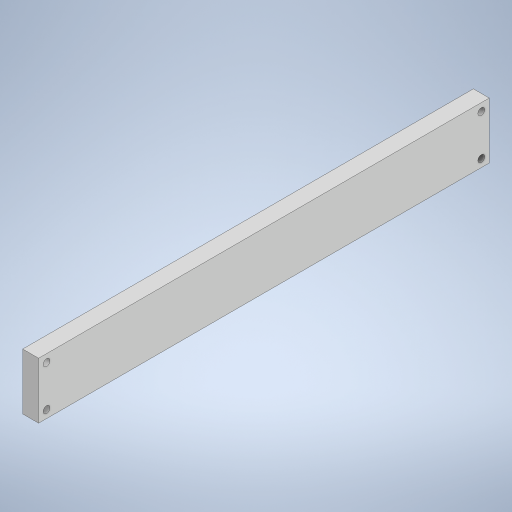
# Autodesk Inventor part: Mold_sideWall
Saved by Autodesk Inventor 2024 (Build 280153000, 153)
## iProperties
Created: 2024-09-09
Part Number: Mold_sideWall
Material: Generic
Document SubType Name: Modeling
Designer: Bruger
Density: 1 g/cm^3
Appearance: Default
Author: Bruger
Autodesk Inventor part; units mm, degrees
ref_plane "YZ Plane" through (0, 0, 0) normal (1, 0, 0) x (0, 1, 0)
ref_plane "XZ Plane" through (0, 0, 0) normal (0, 1, 0) x (-1, 0, 0)
ref_plane "XY Plane" through (0, 0, 0) normal (0, 0, 1) x (1, 0, 0)
sketch "Sketch1" plane through (0, 0, 0) normal (1, 0, 0) x (0, 1, 0)
  line L0 (-12.375, 99.15) -> (12.375, 99.15)
  line L1 (12.375, 99.15) -> (12.375, -99.15)
  line L2 (12.375, -99.15) -> (-12.375, -99.15)
  line L3 (-12.375, -99.15) -> (-12.375, 99.15)
  line L4 (-12.375, 99.15) -> (12.375, -99.15) construction
  line L5 (12.375, 99.15) -> (-12.375, -99.15) construction
  point P0 (0, 0)
  dimension "d0" = 198.3
  dimension "d1" = 24.75
  constraints: 12 end point, 2 midpoint, 2 parallel, 1 horizontal, 1 perpendicular
  measures "d0" distance of L0.end L1.end
  measures "d1" distance between parallel lines of L1 L3
extrude "Extrusion1" add sketch "Sketch1" along normal blind 7
sketch "Sketch2" plane through (7, 0, 0) normal (1, 0, 0) x (0, 0, -1)
  circle A0 centre (-95.65, 8.95) radius 1.5
  line L0 (-99.15, 12.375) -> (-99.15, -12.375) projected
  line L1 (99.15, 12.375) -> (-99.15, 12.375) projected
  line L2 (-113.68, 5.525) -> (-113.68, 12.375)
  point P0 (0, 0)
  dimension "d4" = 3.5
  dimension "d5" = 3.425
  dimension "d13" = 3
  constraints: 2 end point, 1 centre point, 1 perpendicular, 1 point on line
  measures "d4" distance from line of L0 A0.centre
  measures "d5" distance from line of L1 A0.centre
  measures "d13" diameter of A0
hole "Hole1" at (7, 8.95, 95.65) direction (-1, 0, 0) diameter 3 end through all
mirror "Mirror1" about plane through (0, 0, 0) normal (0, 1, 0) of "Hole1"
mirror "Mirror2" about plane through (0, 0, 0) normal (0, 0, 1) of "Hole1", "Mirror1"
sketch "Sketch3" plane through (0, -12.375, -99.15) normal (0, -1, 0) x (1, 0, 0)
  circle A0 centre (3.5, 62.665) radius 1.5
  line L0 (7, 198.3) -> (7, 0) projected
  line L1 (0, 0) -> (7, 0) projected
  point P0 (0, 99.15)
  point P1 (3.5, 0)
  dimension "d14" = 3
  dimension "d15" = 3.5
  dimension "d16" = 62.665
  constraints: 1 centre point, 1 midpoint
  measures "d14" diameter of A0
  measures "d15" distance from line of L0 A0.centre
  measures "d16" distance of point (3.5, 0) A0.centre
hole "Hole2" at (3.5, -12.375, -36.485) direction (0, 1, 0) diameter 3 depth 5 tip angle 118
mirror "Mirror3" about plane through (0, 0, 0) normal (0, 0, 1) of "Hole2"
body "Solid1"
